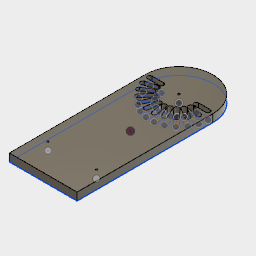
_motor_tips_3D.b541b689-42d2-46c7-8ee2-95b9a4902e00 (Autodesk Fusion 360 design; units mm, degrees)
Autodesk Fusion 360 part; units mm, degrees
sketch "Sketch1" plane through (0, 0, 0) normal (0, 1, 0) x (1, 0, 0)
  line L0 (-17.5, 25) -> (-17.5, -25)
  line L1 (17.5, -25) -> (17.5, 25)
  circle A0 centre (0, 25) radius 0.5
  arc A1 (17.5, 25) -> (-17.5, 25) centre (0, 25) ccw
  line L2 (-15, 23.85) -> (-9, 23.85)
  arc A2 (-9, 23.85) -> (-9, 26.15) centre (-9, 25) ccw
  line L3 (-9, 26.15) -> (-15, 26.15)
  arc A3 (-15, 26.15) -> (-15, 23.85) centre (-15, 25) ccw
  line L4 (-15, 25) -> (-9, 25) construction
  circle A4 centre (-12.5, -30) radius 0.5
  circle A5 centre (12.5, -30) radius 0.5
  line L5 (-17.5, -25) -> (-17.5, -45)
  line L6 (-17.5, -45) -> (17.5, -45)
  line L7 (17.5, -25) -> (17.5, -45)
  arc A6 (-14.7164, 21.8774) -> (-14.0684, 19.6706) centre (-14.3924, 20.774) ccw
  arc A7 (-8.3114, 21.361) -> (-8.9594, 23.5678) centre (-8.6354, 22.4644) ccw
  line L8 (-14.0684, 19.6706) -> (-8.3114, 21.361)
  line L9 (-8.9594, 23.5678) -> (-14.7164, 21.8774)
  line L10 (-14.3924, 20.774) -> (-8.6354, 22.4644) construction
  arc A8 (-13.2405, 17.8578) -> (-11.9971, 15.9229) centre (-12.6188, 16.8904) ccw
  arc A9 (-6.9495, 19.1668) -> (-8.193, 21.1017) centre (-7.5713, 20.1342) ccw
  line L11 (-11.9971, 15.9229) -> (-6.9495, 19.1668)
  line L12 (-8.193, 21.1017) -> (-13.2405, 17.8578)
  line L13 (-12.6188, 16.8904) -> (-7.5713, 20.1342) construction
  arc A10 (-10.692, 14.4168) -> (-8.9538, 12.9107) centre (-9.8229, 13.6638) ccw
  arc A11 (-5.0246, 17.4452) -> (-6.7629, 18.9513) centre (-5.8937, 18.1983) ccw
  line L14 (-8.9538, 12.9107) -> (-5.0246, 17.4452)
  line L15 (-6.7629, 18.9513) -> (-10.692, 14.4168)
  line L16 (-9.8229, 13.6638) -> (-5.8937, 18.1983) construction
  arc A12 (-7.2773, 11.8332) -> (-5.1851, 10.8778) centre (-6.2312, 11.3555) ccw
  arc A13 (-2.6927, 16.3356) -> (-4.7848, 17.291) centre (-3.7387, 16.8133) ccw
  line L17 (-5.1851, 10.8778) -> (-2.6927, 16.3356)
  line L18 (-4.7848, 17.291) -> (-7.2773, 11.8332)
  line L19 (-6.2312, 11.3555) -> (-3.7387, 16.8133) construction
  arc A14 (-3.273, 10.3163) -> (-0.9964, 9.989) centre (-2.1347, 10.1527) ccw
  arc A15 (-0.1425, 15.9279) -> (-2.4191, 16.2553) centre (-1.2808, 16.0916) ccw
  line L20 (-0.9964, 9.989) -> (-0.1425, 15.9279)
  line L21 (-2.4191, 16.2553) -> (-3.273, 10.3163)
  line L22 (-2.1347, 10.1527) -> (-1.2808, 16.0916) construction
  arc A16 (0.9964, 9.989) -> (3.273, 10.3163) centre (2.1347, 10.1527) ccw
  arc A17 (2.4191, 16.2553) -> (0.1425, 15.9279) centre (1.2808, 16.0916) ccw
  line L23 (3.273, 10.3163) -> (2.4191, 16.2553)
  line L24 (0.1425, 15.9279) -> (0.9964, 9.989)
  line L25 (2.1347, 10.1527) -> (1.2808, 16.0916) construction
  arc A18 (5.1851, 10.8778) -> (7.2773, 11.8332) centre (6.2312, 11.3555) ccw
  arc A19 (4.7848, 17.291) -> (2.6927, 16.3356) centre (3.7387, 16.8133) ccw
  line L26 (7.2773, 11.8332) -> (4.7848, 17.291)
  line L27 (2.6927, 16.3356) -> (5.1851, 10.8778)
  line L28 (6.2312, 11.3555) -> (3.7387, 16.8133) construction
  arc A20 (8.9538, 12.9107) -> (10.692, 14.4168) centre (9.8229, 13.6638) ccw
  arc A21 (6.7629, 18.9513) -> (5.0246, 17.4452) centre (5.8937, 18.1983) ccw
  line L29 (10.692, 14.4168) -> (6.7629, 18.9513)
  line L30 (5.0246, 17.4452) -> (8.9538, 12.9107)
  line L31 (9.8229, 13.6638) -> (5.8937, 18.1983) construction
  arc A22 (11.9971, 15.9229) -> (13.2405, 17.8578) centre (12.6188, 16.8904) ccw
  arc A23 (8.193, 21.1017) -> (6.9495, 19.1668) centre (7.5713, 20.1342) ccw
  line L32 (13.2405, 17.8578) -> (8.193, 21.1017)
  line L33 (6.9495, 19.1668) -> (11.9971, 15.9229)
  line L34 (12.6188, 16.8904) -> (7.5713, 20.1342) construction
  arc A24 (14.0684, 19.6706) -> (14.7164, 21.8774) centre (14.3924, 20.774) ccw
  arc A25 (8.9594, 23.5678) -> (8.3114, 21.361) centre (8.6354, 22.4644) ccw
  line L35 (14.7164, 21.8774) -> (8.9594, 23.5678)
  line L36 (8.3114, 21.361) -> (14.0684, 19.6706)
  line L37 (14.3924, 20.774) -> (8.6354, 22.4644) construction
  arc A26 (15, 23.85) -> (15, 26.15) centre (15, 25) ccw
  arc A27 (9, 26.15) -> (9, 23.85) centre (9, 25) ccw
  line L38 (15, 26.15) -> (9, 26.15)
  line L39 (9, 23.85) -> (15, 23.85)
  line L40 (15, 25) -> (9, 25) construction
  dimension "d1" = 50
  dimension "d2" = 35
  dimension "d4" = 1
  dimension "d7" = 15
  dimension "d31" = 2.3
  dimension "d45" = 1
  dimension "d46" = 1
  dimension "d49" = 5
  dimension "d50" = 5
  dimension "d52" = 20
  dimension "d54" = 15
  dimension "d55" = 15
  dimension "d58" = 6
  dimension "d62" = 180
  measures "d1" distance of L0.start L0.end
  measures "d2" distance of L0.end L1.start
  measures "d4" diameter of A0
  measures "d7" distance of A0.centre A3.centre
  measures "d31" diameter of A2
  measures "d45" diameter of A4
  measures "d46" diameter of A5
  measures "d49" distance of L0 A4.centre
  measures "d50" distance of L1 A5.centre
  measures "d52" distance of L0.end L5.end
  measures "d54" distance of A4.centre L6
  measures "d55" distance of A5.centre L6
  measures "d58" distance of A3.centre A2.centre
extrude "Extrude4" add sketch "Sketch1" along normal blind 4
